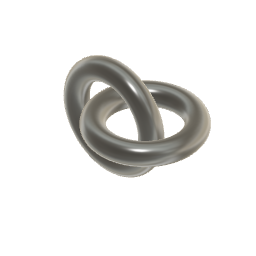
Print v1 (Autodesk Fusion 360 design; units mm, degrees)
Autodesk Fusion 360 part; units mm, degrees
torus "TorusPrimitive1" add centre line diameter 40 section diameter 10 placed x (1, 0, 0) y (0, 1, 0) z (0, 0, 1) at (76.5429, 40.4907, 0) makes body 1
torus "TorusPrimitive2" add centre line diameter 40 section diameter 10 placed x (1, 0, 0) y (0, 0, -1) z (0, 1, 0) at (63.4941, 0, 1.3601) separate body makes body 2
move_body "MoveFace1" bodies 2 to x (1, 0, 0) y (0, 1, 0) z (0, 0, 1) at (-5.3527, 42.1676, -7.9368) on bodies 2
